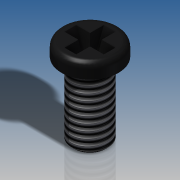
# Autodesk Inventor part: u9013-Black
Saved by Autodesk Inventor 2016 (Build 200138000, 138)
## iProperties
Created: 2015-08-26
Part Number: u9013-Black
Material: Steel
Document SubType Name: Modeling
Designer: D. Kohfeld
Mass: 0.261935 g
Surface Area: 0.822698 cm^2
Volume: 0.0333675 cm^3
Density: 7.85 g/cm^3
Appearance: Black
Author: D. Kohfeld
Autodesk Inventor part; units mm, degrees
ref_plane "YZ Plane" through (0, 0, 0) normal (1, 0, 0) x (0, 1, 0)
ref_plane "XZ Plane" through (0, 0, 0) normal (0, 1, 0) x (-1, 0, 0)
ref_plane "XY Plane" through (0, 0, 0) normal (0, 0, 1) x (1, 0, 0)
sketch "Sketch2" plane through (0, 0, 0) normal (0, 0, 1) x (1, 0, 0)
  line L0 (1.96, 0) -> (1.25, 0)
  line L1 (1.25, 0) -> (1.25, -4.8)
  line L2 (1.25, -4.8) -> (1.05, -5)
  line L3 (1.05, -5) -> (0, -5)
  line L4 (0, -5) -> (0, 1)
  line L5 (0, 1) -> (1.56, 1)
  arc A0 (1.96, 0.6) -> (1.56, 1) centre (1.56, 0.6) ccw
  line L6 (1.96, 0.6) -> (1.96, 0)
  line L7 (1.35, 1) -> (0.6995, -0.1267)
  line L8 (0.6995, -0.1267) -> (0, -0.25)
  line L9 (0, -0.25) -> (-0.6995, -0.1267)
  line L10 (-0.6995, -0.1267) -> (-1.35, 1)
  line L11 (-1.35, 1) -> (1.35, 1)
  line L12 (0.6995, -0.1267) -> (0, -1.3383)
  line L13 (-0.6995, -0.1267) -> (0, -1.3383)
  line L14 (0.6995, -0.1267) -> (1.1648, -0.0446)
  line L15 (1.1648, -0.0446) -> (0, -1.3383)
  point P0 (0, 0)
  dimension "d0" = 45
  dimension "d1" = 0.2
  dimension "d2" = 3.92
  dimension "d3" = 1
  dimension "d4" = 0.4
  dimension "d5" = 2.5
  dimension "d6" = 5
  dimension "d8" = 2.7
  dimension "d9" = 1.25
  dimension "d10" = 60
  dimension "d11" = 160
  dimension "d18" = 42
  constraints: 32 end point, 4 horizontal, 4 point on line, 3 collinear, 3 vertical, 2 equal length, 2 horizontal alignment, 2 point on circle, 2 tangent, 1 centre point, 1 midpoint, 1 vertical alignment
  measures "d0" angle of L2 L3
  measures "d1" horizontal distance of L1.end L2.end
  measures "d2" diameter of L6 L4
  measures "d3" distance between parallel lines of L5 L0
  measures "d4" radius of A0
  measures "d5" diameter of L1 L4
  measures "d6" distance between parallel lines of L3 L0
  measures "d8" diameter of L7.start L4
  measures "d9" distance from line of L5 L8.end
  measures "d10" angle of L7 L10
  measures "d11" angle of L9 L8
  measures "d18" angle of L4 L15
revolve "Revolution1" add sketch "Sketch2" angle 360 about axis through (0, -5, 0) along (0, 1, 0) contours L0 L1 L2 L3 L4 L15 L14 L7 L5 A0 L6 | L7 L8 L4 L5 | L12 L4 L8 | L14 L15 L12
extrude "Extrusion1" cut sketch "Sketch2" along normal mid plane 0.8 contours L7 L8 L4 L5 | L4 L9 L10 L11 | L12 L4 L8 | L13 L9 L4
pattern_circular "Circular Pattern1" count 2 over 90 about axis through (0, 0.3, 0) along (0, -1, 0) of "Extrusion1"
revolve "Revolution2" add sketch "Sketch2" angle 360 about axis through (0, -5, 0) along (0, 1, 0) contours L12 L4 L8 | L14 L15 L12
draft "FaceDraft2" angle 8 pull direction (0, 1, 0) faces at (-0.8205, 0.6313, 0.4) (-0.4, 0.6313, 0.8205) (0.8205, 0.6313, 0.4) (0.4, 0.6313, 0.8205) (0.8205, 0.6313, -0.4) (0.4, 0.6313, -0.8205) (-0.4, 0.6313, -0.8205) (-0.8205, 0.6313, -0.4) fixed edges at (-0.875, 1, 0.4) (-0.4, 1, 0.875) (0.875, 1, 0.4) (0.4, 1, 0.875) (0.875, 1, -0.4) (0.4, 1, -0.875) (-0.4, 1, -0.875) (-0.875, 1, -0.4)
thread "Thread1" size "M2.5x0.45" class "6g" standard "ANSI Metric M Profile" full length
body "Solid1"
